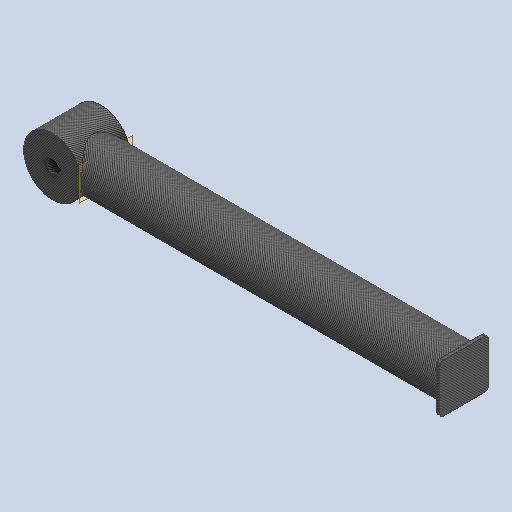
# Autodesk Inventor part: czlon 3
Saved by Autodesk Inventor 2023 (Build 270158000, 158)
## iProperties
Created: 2023-04-13
Part Number: czlon 3
Material: CFRP — polimer wzmocniony włóknem szklanym
Document SubType Name: Modeling
Designer: krzys
Density: 1.43 g/cm^3
Appearance: Włókno węglowe
Mass: 960.186 g
Surface Area: 3325.08 cm^2
Volume: 671.459 cm^3
Author: krzys
Autodesk Inventor part; units mm, degrees
ref_plane "XZ Plane" through (0, 0, 0) normal (0, 1, 0) x (-1, 0, 0)
ref_plane "XY Plane" through (0, 0, 0) normal (0, 0, 1) x (1, 0, 0)
sketch "Szkic3" plane through (0, 0, 0) normal (0, 0, 1) x (1, 0, 0)
  circle A0 centre (0, 0) radius 45
  circle A1 centre (0, 0) radius 41
  circle A2 centre (0, 0) radius 15
  arc A3 (9.5394, 3) -> (9.5394, -3) centre (0, 0) ccw
  line L0 (13, 3) -> (9.5394, 3)
  line L1 (9.5394, -3) -> (13, -3)
  line L2 (13, -3) -> (13, 3)
  line L3 (13, 3) -> (10, 0) construction
  line L4 (10, 0) -> (13, -3) construction
  dimension "d0" = 90
  dimension "d1" = 82
  dimension "d3" = 30
  dimension "d19" = 20
  constraints: 10 end point, 4 centre point, 3 coincident, 2 point on circle, 1 horizontal, 1 parallel
  measures "d0" diameter of A0
  measures "d1" diameter of A1
  measures "d3" diameter of A2
  measures "d19" diameter of A3
extrude "Wyciągnięcie proste1" add sketch "Szkic3" along normal mid plane 75 contours A0 | A1 | A2 | L0 L2 L1 A3
extrude "Wyciągnięcie proste2" cut sketch "Szkic3" along normal mid plane 68 contours A1
ref_plane "Płaszczyzna konstrukcyjna1" through (45, 0, 0) normal (1, 0, 0) x (0, 1, 0)
sketch "Szkic4" plane through (45, 0, 0) normal (1, 0, 0) x (0, 1, 0)
  circle A0 centre (0, 0) radius 37.5
  circle A1 centre (0, 0) radius 33.5
  dimension "d10" = 67
  constraints: 2 centre point, 2 coincident
  measures "d10" diameter of A1
extrude "Wyciągnięcie proste3" add sketch "Szkic4" along normal blind 550 and the other way blind 20
sketch "Szkic5" plane through (595, 0, 0) normal (1, 0, 0) x (0, 0, -1)
  line L0 (-37.5, 37.5) -> (37.5, 37.5)
  line L1 (37.5, 37.5) -> (37.5, -37.5)
  line L2 (37.5, -37.5) -> (-37.5, -37.5)
  line L3 (-37.5, -37.5) -> (-37.5, 37.5)
  line L4 (-37.5, 37.5) -> (37.5, -37.5) construction
  line L5 (37.5, 37.5) -> (-37.5, -37.5) construction
  point P0 (0, 0)
  point P1 (37.5, 0)
  dimension "d15" = 75
  constraints: 12 end point, 2 midpoint, 2 parallel, 1 horizontal, 1 perpendicular
  measures "d15" distance of L0.end L1.end
extrude "Wyciągnięcie proste4" add sketch "Szkic5" along normal blind 5
fillet "Zaokrąglenie1" radius 5 4 edges at (597.5, 37.5, 37.5) (597.5, 37.5, -37.5) (597.5, -37.5, 37.5) (597.5, -37.5, -37.5)
extrude "Wyciągnięcie proste5" cut sketch "Szkic3" along normal mid plane 75 contours L0 L2 L1 A3
